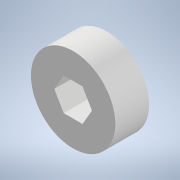
# Autodesk Inventor part: Rodamiento_Ejes
Saved by Autodesk Inventor 2022 (Build 260153000, 153)
## iProperties
Created: 2022-02-21
Part Number: Rodamiento_Ejes
Material: Generic
Document SubType Name: Modeling
Designer: katha
Density: 1 g/cm^3
Appearance: Default
Author: katha
Autodesk Inventor part; units mm, degrees
ref_plane "YZ Plane" through (0, 0, 0) normal (1, 0, 0) x (0, 1, 0)
ref_plane "XZ Plane" through (0, 0, 0) normal (0, 1, 0) x (-1, 0, 0)
ref_plane "XY Plane" through (0, 0, 0) normal (0, 0, 1) x (1, 0, 0)
sketch "Sketch1" plane through (0, 0, 0) normal (0, 0, 1) x (1, 0, 0)
  line L0 (-1.6732, 2.8981) -> (1.6732, 2.8981) projected
  line L1 (-3.3464, 0) -> (-1.6732, 2.8981) projected
  line L2 (-1.6732, -2.8981) -> (-3.3464, 0) projected
  line L3 (1.6732, -2.8981) -> (-1.6732, -2.8981) projected
  line L4 (3.3464, 0) -> (1.6732, -2.8981) projected
  line L5 (1.6732, 2.8981) -> (3.3464, 0) projected
  circle A0 centre (0, 0) radius 7.5
  dimension "d0" = 15
  constraints: 1 centre point, 1 coincident
  measures "d0" diameter of A0
extrude "Extrusion1" add sketch "Sketch1" against normal blind 6
body "Solid1"
